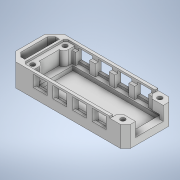
# Autodesk Inventor part: Case_main
Saved by Autodesk Inventor 2020 (Build 240168000, 168)
## iProperties
Created: 2022-03-19
Part Number: Case_main
Material: Типовые
Document SubType Name: Modeling
Designer: NoName
Density: 1 g/cm^3
Appearance: По умолчанию
Author: NoName
Autodesk Inventor part; units mm, degrees
ref_plane "YZ Plane" through (0, 0, 0) normal (1, 0, 0) x (0, 1, 0)
ref_plane "XZ Plane" through (0, 0, 0) normal (0, 1, 0) x (-1, 0, 0)
ref_plane "XY Plane" through (0, 0, 0) normal (0, 0, 1) x (1, 0, 0)
sketch "Эскиз1" plane through (0, 0, 0) normal (0, 1, 0) x (-1, 0, 0)
  line L0 (0, 0) -> (0, -18.4)
  line L1 (0, -18.4) -> (39.8, -18.4)
  line L2 (39.8, -18.4) -> (39.8, -15.55)
  arc A0 (41.8, -13.55) -> (39.8, -15.55) centre (41.8, -15.55) ccw
  line L3 (41.8, -15.55) -> (41.8, -13.55) construction
  line L4 (41.8, -15.55) -> (39.8, -15.55) construction
  line L5 (41.8, -13.55) -> (41.8, -4.85)
  line L6 (41.8, -9.2) -> (0, -9.2)
  line L7 (0, 0) -> (39.8, 0)
  line L8 (39.8, 0) -> (39.8, -2.85)
  arc A1 (39.8, -2.85) -> (41.8, -4.85) centre (41.8, -2.85) ccw
  line L9 (41.8, -2.85) -> (41.8, -4.85) construction
  line L10 (41.8, -2.85) -> (39.8, -2.85) construction
  line L11 (45.8, -19.6) -> (0.4, -19.6)
  line L12 (45.8, 1.2) -> (0.4, 1.2)
  line L13 (49.8, -15.6) -> (49.8, -2.8)
  line L14 (44.8, -16.7) -> (44.8, -1.7)
  line L15 (48.3, -14.9787) -> (48.3, -3.4213)
  line L16 (5.1, -18.4) -> (5.1, -17.1)
  line L17 (5.1, -17.1) -> (0, -17.1)
  line L18 (5.1, 0) -> (5.1, -1.3)
  line L19 (5.1, -1.3) -> (0, -1.3)
  line L20 (0.4, -19.6) -> (-1.6, -17.6)
  line L21 (-1.6, -17.6) -> (-1.6, -0.8)
  line L22 (-1.6, -0.8) -> (0.4, 1.2)
  line L23 (45.8, 1.2) -> (49.8, -2.8)
  line L24 (49.8, -15.6) -> (45.8, -19.6)
  line L25 (48.3, -14.9787) -> (46.5787, -16.7)
  line L26 (46.5787, -16.7) -> (44.8, -16.7)
  line L27 (48.3, -3.4213) -> (46.5787, -1.7)
  line L28 (46.5787, -1.7) -> (44.8, -1.7)
  point P0 (5.1, 0)
  point P1 (0, -1.3)
  point P2 (44.8, -9.2)
  point P3 (48.3, -9.2)
  point P4 (49.8, -9.2)
  dimension "d1" = 41.8
  dimension "d3" = 2
  dimension "d4" = 12.7
  dimension "d8" = 18.4
  dimension "d12" = 3.5
  dimension "d32" = 20.8
  dimension "d34" = 5.1
  dimension "d35" = 15.8
  dimension "d41" = 135
  dimension "d42" = 1.6
  dimension "d43" = 2
  dimension "d65" = 8
  dimension "d66" = 1.5
  dimension "d67" = 15
  dimension "d68" = 1.5
  dimension "d69" = 4
  constraints: 59 end point, 13 symmetric about line, 7 vertical, 6 perpendicular, 5 midpoint, 4 point on circle, 3 horizontal alignment, 2 centre point, 2 point on line, 1 horizontal, 1 parallel, 1 tangent, 1 other
  measures "d1" distance between parallel lines of L0 L5
  measures "d3" distance between parallel lines of L5 L8
  measures "d4" distance of L9.start L3.start
  measures "d8" distance between parallel lines of L7 L1
  measures "d12" distance between parallel lines of L15 L14
  measures "d32" distance between parallel lines of L12 L11
  measures "d34" distance between parallel lines of L0 L16
  measures "d35" distance between parallel lines of L19 L17
  measures "d41" angle of L12 L22
  measures "d42" distance between parallel lines of L0 L21
  measures "d43" horizontal distance of L21.end L12.end
  measures "d65" distance between parallel lines of L5 L13
  measures "d66" distance between parallel lines of L13 L15
  measures "d67" distance between parallel lines of L28 L26
  measures "d68" distance between parallel lines of L24 L25
  measures "d69" distance from line of L5 L11.start
extrude "Выдавливание1" add sketch "Эскиз1" along normal blind 6 contours L7 L18 L19 L0 | L17 L16 L1 L0 | L11 L20 L21 L22 L12 L23 L13 L24
sketch "Эскиз2" plane through (0, 0, 0) normal (0, -1, 0) x (1, 0, 0)
  line L0 (-0.4, -19.6) -> (-45.8, -19.6) projected
  line L1 (-45.8, 1.2) -> (-0.4, 1.2) projected
  line L2 (-49.8, -15.6) -> (-49.8, -2.8) projected
  line L3 (-41.8, -4.85) -> (-41.8, -13.55) projected
  arc A0 (-41.8, -4.85) -> (-39.8, -2.85) centre (-41.8, -2.85) ccw projected
  line L4 (-39.8, 0) -> (-39.8, -2.85) projected
  line L5 (-5.1, 0) -> (-39.8, 0) projected
  line L6 (0, -17.1) -> (0, -1.3) projected
  line L7 (-39.8, -18.4) -> (-5.1, -18.4) projected
  line L8 (-39.8, -15.55) -> (-39.8, -18.4) projected
  arc A1 (-39.8, -15.55) -> (-41.8, -13.55) centre (-41.8, -15.55) ccw projected
  line L9 (-39.8, -15.55) -> (-39.8, -18.4) projected
  line L10 (-39.8, -18.4) -> (-5.1, -18.4) projected
  line L11 (-38.8, -16.5) -> (-1.5, -16.5)
  line L12 (-1.5, -16.5) -> (-1.5, -1.9)
  line L13 (-1.5, -1.9) -> (-38.8, -1.9)
  line L14 (-38.8, -1.9) -> (-38.8, -16.5)
  line L15 (-5.1, -1.3) -> (-5.1, 0) projected
  line L16 (0, -1.3) -> (-5.1, -1.3) projected
  line L17 (-5.1, -17.1) -> (0, -17.1) projected
  line L18 (-5.1, -18.4) -> (-5.1, -17.1) projected
  line L19 (1.6, -17.6) -> (-0.4, -19.6) projected
  line L20 (1.6, -0.8) -> (1.6, -17.6) projected
  line L21 (-0.4, 1.2) -> (1.6, -0.8) projected
  line L22 (-49.8, -2.8) -> (-45.8, 1.2) projected
  line L23 (-45.8, -19.6) -> (-49.8, -15.6) projected
  line L24 (-48.3, -3.4213) -> (-48.3, -14.9787) projected
  line L25 (-46.5787, -1.7) -> (-48.3, -3.4213) projected
  line L26 (-44.8, -1.7) -> (-46.5787, -1.7) projected
  line L27 (-44.8, -16.7) -> (-44.8, -1.7) projected
  line L28 (-46.5787, -16.7) -> (-44.8, -16.7) projected
  line L29 (-48.3, -14.9787) -> (-46.5787, -16.7) projected
  point P0 (0, -18.2)
  point P1 (-41.8, -9.2)
  point P2 (-38.8, -9.2)
  dimension "d17" = 1.5
  dimension "d18" = 3
  dimension "d33" = 14.6
  constraints: 8 end point, 2 midpoint, 2 parallel, 1 horizontal, 1 horizontal alignment, 1 perpendicular, 1 other
  measures "d17" distance between parallel lines of L6 L12
  measures "d18" distance between parallel lines of L3 L14
  measures "d33" distance between parallel lines of L13 L11
extrude "Выдавливание2" add sketch "Эскиз2" along normal blind 1.8 contours L0 L23 L2 L22 L1 L21 L20 L19 | A0 L4 L5 L15 L16 L6 L17 L18 L7 L8 A1 L3
sketch "Эскиз3" plane through (0, -1.8, 0) normal (0, -1, 0) x (1, 0, 0)
  line L0 (-0.4, 1.2) -> (-45.8, 1.2) projected
  line L1 (-49.8, -2.8) -> (-49.8, -15.6) projected
  line L2 (-45.8, -19.6) -> (-0.4, -19.6) projected
  line L3 (-1.5, -1.9) -> (-1.5, -16.5) projected
  line L4 (-1.5, -16.5) -> (-38.8, -16.5) projected
  line L5 (-38.8, -16.5) -> (-38.8, -1.9) projected
  line L6 (-38.8, -1.9) -> (-1.5, -1.9) projected
  line L7 (-0.4, -19.6) -> (1.6, -17.6) projected
  line L8 (1.6, -17.6) -> (1.6, -0.8) projected
  line L9 (1.6, -0.8) -> (-0.4, 1.2) projected
  line L10 (-45.8, 1.2) -> (-49.8, -2.8) projected
  line L11 (-49.8, -15.6) -> (-45.8, -19.6) projected
  line L12 (-48.3, -14.9787) -> (-48.3, -3.4213) projected
  line L13 (-48.3, -3.4213) -> (-46.5787, -1.7) projected
  line L14 (-46.5787, -1.7) -> (-44.8, -1.7) projected
  line L15 (-44.8, -1.7) -> (-44.8, -16.7) projected
  line L16 (-44.8, -16.7) -> (-46.5787, -16.7) projected
  line L17 (-46.5787, -16.7) -> (-48.3, -14.9787) projected
  point P0 (0, 0)
extrude "Выдавливание3" add sketch "Эскиз3" along normal blind 1.2 contours L9 L8 L7 L2 L11 L1 L10 L0 | L3 L4 L5 L6
sketch "Эскиз5" plane through (-45.8, 6, 1.2) normal (0, 0, 1) x (1, 0, 0)
  line L0 (7.6, 0) -> (13.6, 0)
  line L1 (13.6, 0) -> (13.6, -5)
  line L2 (13.6, -5) -> (7.6, -5)
  line L3 (7.6, -5) -> (7.6, 0)
  line L4 (0, 0) -> (45.4, 0) projected
  line L5 (4, -6) -> (4, 0) projected
  point P0 (45.8, -6)
  point P1 (46.5, 0)
  dimension "d27" = 6
  dimension "d28" = 5
  dimension "d29" = 3.6
  constraints: 8 end point, 2 parallel, 1 horizontal, 1 perpendicular, 1 point on line
  measures "d27" distance between parallel lines of L3 L1
  measures "d28" distance between parallel lines of L0 L2
  measures "d29" distance between parallel lines of L5 L3
extrude "Выдавливание5" cut sketch "Эскиз5" against normal through all
pattern_linear "Прямоуг.массив1" count 4 spacing 8.5 along (1, 0, 0) of "Выдавливание5"
sketch "Эскиз6" plane through (0, 0, 0) normal (0, 1, 0) x (1, 0, 0)
  line L0 (-5.1, 0) -> (-39.8, 0) projected
  line L1 (-15.2, 0) -> (-12.7, 0)
  line L2 (-12.7, 0) -> (-12.7, 1.3)
  line L3 (-12.7, 1.3) -> (-15.2, 1.3)
  line L4 (-15.2, 1.3) -> (-15.2, 0)
  line L5 (-23.7, 0) -> (-21.2, 0)
  line L6 (-21.2, 0) -> (-21.2, 1.3)
  line L7 (-21.2, 1.3) -> (-23.7, 1.3)
  line L8 (-23.7, 1.3) -> (-23.7, 0)
  line L9 (-32.2, 0) -> (-29.7, 0)
  line L10 (-29.7, 0) -> (-29.7, 1.3)
  line L11 (-29.7, 1.3) -> (-32.2, 1.3)
  line L12 (-32.2, 1.3) -> (-32.2, 0)
  line L13 (-38.2, 0) -> (-39.8, 0)
  line L14 (-39.8, 0) -> (-39.8, 1.3)
  line L15 (-39.8, 1.3) -> (-38.2, 1.3)
  line L16 (-38.2, 1.3) -> (-38.2, 0)
  line L17 (-5.1, 0) -> (-6.7, 0) projected
  line L18 (-5.1, 0) -> (-39.8, 0) projected
  line L19 (-38.2, 0) -> (-39.8, 0) projected
  line L20 (-38.2, 0) -> (-32.2, 0) projected
  line L21 (0, 1.3) -> (-5.1, 1.3) projected
  line L22 (-6.7, 0) -> (-5.1, 0)
  line L23 (-5.1, 0) -> (-5.1, 1.3)
  line L24 (-5.1, 1.3) -> (-6.7, 1.3)
  line L25 (-6.7, 1.3) -> (-6.7, 0)
  line L26 (-41.8, 4.85) -> (-41.8, 13.55) projected
  line L27 (-41.8, 9.2) -> (-1.5, 9.2)
  line L28 (-5.1, 18.4) -> (-39.8, 18.4)
  line L29 (-15.2, 18.4) -> (-12.7, 18.4)
  line L30 (-12.7, 18.4) -> (-12.7, 17.1)
  line L31 (-12.7, 17.1) -> (-15.2, 17.1)
  line L32 (-15.2, 17.1) -> (-15.2, 18.4)
  line L33 (-23.7, 18.4) -> (-21.2, 18.4)
  line L34 (-21.2, 18.4) -> (-21.2, 17.1)
  line L35 (-21.2, 17.1) -> (-23.7, 17.1)
  line L36 (-23.7, 17.1) -> (-23.7, 18.4)
  line L37 (-32.2, 18.4) -> (-29.7, 18.4)
  line L38 (-29.7, 18.4) -> (-29.7, 17.1)
  line L39 (-29.7, 17.1) -> (-32.2, 17.1)
  line L40 (-32.2, 17.1) -> (-32.2, 18.4)
  line L41 (-38.2, 18.4) -> (-39.8, 18.4)
  line L42 (-39.8, 18.4) -> (-39.8, 17.1)
  line L43 (-39.8, 17.1) -> (-38.2, 17.1)
  line L44 (-38.2, 17.1) -> (-38.2, 18.4)
  line L45 (-5.1, 18.4) -> (-6.7, 18.4)
  line L46 (-5.1, 18.4) -> (-39.8, 18.4)
  line L47 (-38.2, 18.4) -> (-39.8, 18.4)
  line L48 (-38.2, 18.4) -> (-32.2, 18.4)
  line L49 (-29.7, 18.4) -> (-32.2, 18.4)
  line L50 (-29.7, 18.4) -> (-23.7, 18.4)
  line L51 (-21.2, 18.4) -> (-23.7, 18.4)
  line L52 (-21.2, 18.4) -> (-15.2, 18.4)
  line L53 (-12.7, 18.4) -> (-15.2, 18.4)
  line L54 (-12.7, 18.4) -> (-6.7, 18.4)
  line L55 (0, 17.1) -> (-5.1, 17.1)
  line L56 (-6.7, 18.4) -> (-5.1, 18.4)
  line L57 (-5.1, 18.4) -> (-5.1, 17.1)
  line L58 (-5.1, 17.1) -> (-6.7, 17.1)
  line L59 (-6.7, 17.1) -> (-6.7, 18.4)
  line L60 (-1.5, 1.9) -> (-1.5, 16.5) projected
  line L61 (-29.7, 0) -> (-32.2, 0) projected
  line L62 (-29.7, 0) -> (-23.7, 0) projected
  line L63 (-21.2, 0) -> (-23.7, 0) projected
  line L64 (-21.2, 0) -> (-15.2, 0) projected
  line L65 (-12.7, 0) -> (-15.2, 0) projected
  line L66 (-12.7, 0) -> (-6.7, 0) projected
  point P0 (0, 0)
  point P1 (0, 18.4)
  point P2 (-6.7, 18.4)
  point P3 (-21.2, 18.4)
  point P4 (-29.7, 18.4)
  point P5 (-6.7, 0)
  point P6 (-12.7, 0)
  point P7 (-21.2, 0)
  point P8 (-29.7, 0)
  constraints: 106 end point, 29 symmetric about line, 10 parallel, 10 point on line, 6 horizontal, 5 perpendicular, 4 horizontal alignment, 2 midpoint
extrude "Выдавливание6" add sketch "Эскиз6" along normal blind 5
sketch "Эскиз7" plane through (1.6, 6, -0.8) normal (1, 0, 0) x (0, 0, -1)
  line L0 (15.9, 0) -> (0.9, 0) projected
  line L1 (14.4, 0) -> (2.4, 0)
  line L2 (2.4, 0) -> (2.4, -6)
  line L3 (2.4, -6) -> (14.4, -6)
  line L4 (14.4, -6) -> (14.4, 0)
  point P0 (-0.8, -6)
  point P1 (16.5, 0)
  point P2 (-0.5, 0)
  point P3 (8.4, 0)
  point P4 (2.4, 0)
  dimension "d44" = 12
  dimension "d45" = 6
  constraints: 8 end point, 2 midpoint, 2 parallel, 1 horizontal, 1 perpendicular, 1 point on line
  measures "d44" distance between parallel lines of L4 L2
  measures "d45" distance between parallel lines of L3 L0
extrude "Выдавливание7" cut sketch "Эскиз7" against normal up to next
ref_plane "РабПлоскость1" through (0, 1.8, 0) normal (0, 1, 0) x (1, 0, 0)
sketch "Эскиз8" plane through (0, 1.8, 0) normal (0, 1, 0) x (1, 0, 0)
  line L0 (0, 17.1) -> (0, 15.2) projected
  line L1 (0, 17.1) -> (-5.1, 17.1)
  line L2 (0, 15.2) -> (0, 17.1)
  line L3 (-41.8, 4.85) -> (-41.8, 13.55) projected
  line L4 (-41.8, 9.2) -> (1.6, 9.2)
  line L5 (1.6, 15.2) -> (1.6, 3.2) projected
  line L6 (-5.1, 17.1) -> (-3.2, 15.2)
  line L7 (-3.2, 15.2) -> (0, 15.2)
  line L8 (0, 17.1) -> (-6.7, 17.1) projected
  line L9 (0, 1.3) -> (0, 3.2)
  line L10 (0, 1.3) -> (-5.1, 1.3)
  line L11 (0, 3.2) -> (0, 1.3)
  line L12 (-5.1, 1.3) -> (-3.2, 3.2)
  line L13 (-3.2, 3.2) -> (0, 3.2)
  point P0 (0, 0)
  point P1 (-5.1, 17.1)
  dimension "d49" = 45
  constraints: 20 end point, 5 symmetric about line, 2 midpoint, 2 point on line, 1 horizontal, 1 parallel
  measures "d49" angle of L1 L6
extrude "Выдавливание8" add sketch "Эскиз8" along normal up to surface (4.2 mm away)
sketch "Эскиз10" plane through (0, 6, 0) normal (0, 1, 0) x (1, 0, 0)
  line L0 (-41.8, 4.85) -> (-41.8, 13.55) projected
  line L1 (-41.8, 9.2) -> (-1.5, 9.2)
  line L2 (-1.5, 1.9) -> (-1.5, 16.5) projected
  line L3 (-44.8, 16.7) -> (-44.8, 1.7) projected
  line L4 (1.6, 15.2) -> (1.6, 17.6) projected
  point P0 (0, 0)
  point P1 (-41.8875, 16.2)
  point P2 (-41.8875, 2.2)
  point P3 (-1.9, 17.2)
  point P4 (-1.9, 1.2)
  point P5 (-44.8, 17.7)
  point P6 (-44.8, 0.7)
  dimension "d59" = 16
  dimension "d60" = 14
  dimension "d62" = 3.5
  dimension "d63" = 40
  constraints: 2 end point, 2 midpoint, 2 symmetric about line
  measures "d59" distance of point (-1.9, 1.2) point (-1.9, 17.2)
  measures "d60" distance of point (-41.887, 2.2) point (-41.887, 16.2)
  measures "d62" distance from line of L4 point (-1.9, 17.2)
  measures "d63" distance of point (-1.9, 17.2) point (-41.887, 16.2)
hole "Отверстие1" at (-41.8875, 6, -16.2) at (-41.8875, 6, -2.2) at (-1.9, 6, -17.2) at (-1.9, 6, -1.2) direction (0, -1, 0) diameter 2 depth 6
sketch "Эскиз13" plane through (0, 6, 0) normal (0, 1, 0) x (1, 0, 0)
  circle A0 centre (-41.8875, 16.2) radius 1 projected
  circle A1 centre (-41.8875, 2.2) radius 1 projected
  line L0 (-46.5787, 1.7) -> (-48.3, 3.4213) projected
  line L1 (-48.3, 3.4213) -> (-48.3, 14.9787) projected
  line L2 (-48.3, 14.9787) -> (-46.5787, 16.7) projected
  line L3 (-46.5787, 16.7) -> (-44.8, 16.7) projected
  line L4 (-44.8, 16.7) -> (-44.8, 1.7) projected
  line L5 (-44.8, 1.7) -> (-46.5787, 1.7) projected
  line L6 (-49.8, 2.8) -> (-45.8, -1.2) projected
  line L7 (-45.8, -1.2) -> (-38.2, -1.2) projected
  line L8 (-38.2, -1.2) -> (-38.2, 0) projected
  line L9 (-38.2, 0) -> (-39.8, 0) projected
  line L10 (-39.8, 0) -> (-39.8, 2.85) projected
  arc A2 (-39.8, 2.85) -> (-41.8, 4.85) centre (-41.8, 2.85) ccw projected
  line L11 (-41.8, 4.85) -> (-41.8, 13.55) projected
  arc A3 (-41.8, 13.55) -> (-39.8, 15.55) centre (-41.8, 15.55) ccw projected
  line L12 (-39.8, 15.55) -> (-39.8, 18.4) projected
  line L13 (-39.8, 18.4) -> (-38.2, 18.4) projected
  line L14 (-38.2, 18.4) -> (-38.2, 19.6) projected
  line L15 (-38.2, 19.6) -> (-45.8, 19.6) projected
  line L16 (-45.8, 19.6) -> (-49.8, 15.6) projected
  line L17 (-49.8, 15.6) -> (-49.8, 2.8) projected
  line L18 (-39.8, 18.4) -> (-38.2, 18.4) projected
  line L19 (-6.7, 18.4) -> (-12.7, 18.4) projected
  line L20 (-38.2, 18.4) -> (-6.7, 18.4)
  line L21 (-5.1, 18.4) -> (-5.1, 17.1) projected
  line L22 (-6.7, 18.4) -> (-5.1, 18.4)
  line L23 (-5.1, 18.4) -> (-5.1, 19.6)
  line L24 (-0.4, 19.6) -> (-6.7, 19.6) projected
  line L25 (-5.1, 19.6) -> (-38.2, 19.6)
  line L26 (-45.8, 19.6) -> (-0.4, 19.6) projected
  line L27 (-38.2, 0) -> (-39.8, 0) projected
  line L28 (-5.1, 0) -> (-6.7, 0) projected
  line L29 (-38.2, 0) -> (-5.1, 0)
  line L30 (-5.1, 0) -> (-5.1, -1.2)
  line L31 (-0.4, -1.2) -> (-45.8, -1.2) projected
  line L32 (-38.2, -1.2) -> (-38.2, 0) projected
  line L33 (-5.1, -1.2) -> (-38.2, -1.2)
  line L34 (-39.8, 0) -> (-39.8, 1.3) projected
  line L35 (-39.8, 18.4) -> (-42.8, 18.4)
  line L36 (-42.8, 18.4) -> (-43.8, 17.4)
  line L37 (-43.8, 17.4) -> (-43.8, 1)
  line L38 (-43.8, 1) -> (-42.8, 0)
  line L39 (-42.8, 0) -> (-39.8, 0)
  line L40 (-41.8, 4.85) -> (-41.8, 13.55) projected
  line L41 (-41.8, 9.2) -> (-1.5, 9.2)
  line L42 (-1.5, 1.9) -> (-1.5, 16.5) projected
  point P0 (0, 0)
  point P1 (-1.5, 2.1165)
  point P2 (-1.5, 16.2835)
  point P3 (-12.7, 18.4)
  point P4 (-6.7, 0)
  dimension "d71" = 1
  dimension "d72" = 1
  constraints: 26 end point, 5 perpendicular, 4 horizontal, 2 collinear, 2 midpoint, 2 point on line, 1 parallel, 1 other
  measures "d71" distance between parallel lines of L4 L37
  measures "d72" horizontal distance of L35.end L36.end
extrude "Выдавливание9" add sketch "Эскиз13" along normal blind 0.8 contours L17 L16 L15 L14 L13 L35 L36 L37 L38 L39 L9 L8 L7 L6 | L8 L29 L28 L30 L31 | L25 L24 L23 L22 L19 L20 L14
